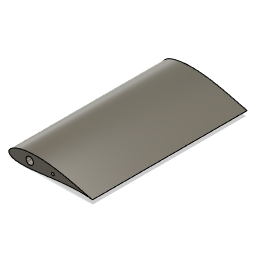
Joukowsky Refactor v1 (Autodesk Fusion 360 design; units mm, degrees)
Autodesk Fusion 360 part; units mm, degrees
sketch "Esquisse2" plane through (0, 0, 0) normal (0, 0, 1) x (1, 0, 0)
  spline S0 degree 5 poles (50, 0) (50, 0) (49.9928, 0.0013) (49.9605, 0.0071) (49.9137, 0.0157) (49.8549, 0.027) (49.7783, 0.0417) (49.6918, 0.0586) (49.6021, 0.0764) (49.5093, 0.0951) (49.4111, 0.1151) (49.3071, 0.1365) (49.1985, 0.159) (49.0867, 0.1824) (48.9721, 0.2067) (48.8543, 0.2319) (48.7333, 0.2579) (48.6092, 0.2848) (48.4821, 0.3126) (48.3526, 0.3411) (48.2206, 0.3703) (48.0864, 0.4002) (47.9499, 0.4309) (47.8111, 0.4622) (47.6702, 0.4942) (47.5272, 0.5268) (47.3822, 0.56) (47.2354, 0.5939) (47.0867, 0.6283) (46.9363, 0.6633) (46.7842, 0.6989) (46.6303, 0.735) (46.4749, 0.7717) (46.3178, 0.8089) (46.1592, 0.8466) (45.9991, 0.8848) (45.8376, 0.9234) (45.6746, 0.9626) (45.5102, 1.0022) (45.3445, 1.0423) (45.1775, 1.0828) (45.0092, 1.1238) (44.8396, 1.1652) (44.6688, 1.207) (44.4967, 1.2492) (44.3235, 1.2918) (44.1492, 1.3348) (43.9737, 1.3782) (43.797, 1.422) (43.6194, 1.4661) (43.4406, 1.5106) (43.2608, 1.5554) (43.08, 1.6006) (42.8981, 1.6461) (42.7153, 1.692) (42.5315, 1.7382) (42.3468, 1.7847) (42.1611, 1.8315) (41.9745, 1.8786) (41.787, 1.926) (41.5986, 1.9736) (41.4094, 2.0216) (41.2192, 2.0699) (41.0283, 2.1184) (40.8365, 2.1671) (40.6439, 2.2162) (40.4505, 2.2654) (40.2564, 2.315) (40.0614, 2.3647) (39.8657, 2.4147) (39.6692, 2.4649) (39.472, 2.5154) (39.2741, 2.566) (39.0754, 2.6169) (38.8761, 2.668) (38.676, 2.7192) (38.4753, 2.7707) (38.2738, 2.8223) (38.0718, 2.8742) (37.869, 2.9262) (37.6656, 2.9784) (37.4616, 3.0307) (37.257, 3.0832) (37.0517, 3.1359) (36.8458, 3.1887) (36.6394, 3.2417) (36.4323, 3.2948) (36.2247, 3.348) (36.0164, 3.4014) (35.8076, 3.4549) (35.5983, 3.5085) (35.3884, 3.5623) (35.1779, 3.6161) (34.9669, 3.6701) (34.7554, 3.7241) (34.5434, 3.7783) (34.3308, 3.8326) (34.1177, 3.8869) (33.9041, 3.9414) (33.6901, 3.9959) (33.4755, 4.0505) (33.2605, 4.1051) (33.0449, 4.1599) (32.8289, 4.2147) (32.6125, 4.2696) (32.3956, 4.3245) (32.1782, 4.3794) (31.9604, 4.4345) (31.7421, 4.4895) (31.5234, 4.5446) (31.3043, 4.5998) (31.0848, 4.6549) (30.8648, 4.7101) (30.6444, 4.7653) (30.4237, 4.8206) (30.2025, 4.8758) (29.9809, 4.9311) (29.7589, 4.9863) (29.5366, 5.0416) (29.3138, 5.0969) (29.0907, 5.1521) (28.8672, 5.2074) (28.6433, 5.2627) (28.4191, 5.3179) (28.1945, 5.3731) (27.9696, 5.4283) (27.7443, 5.4834) (27.5186, 5.5386) (27.2927, 5.5937) (27.0664, 5.6487) (26.8397, 5.7037) (26.6128, 5.7587) (26.3855, 5.8136) (26.1578, 5.8685) (25.9299, 5.9233) (25.7017, 5.9781) (25.4731, 6.0328) (25.2443, 6.0874) (25.0152, 6.142) (24.7857, 6.1965) (24.556, 6.2509) (24.326, 6.3052) (24.0957, 6.3595) (23.8651, 6.4136) (23.6342, 6.4677) (23.4031, 6.5217) (23.1717, 6.5756) (22.9401, 6.6293) (22.7081, 6.683) (22.476, 6.7366) (22.2435, 6.7901) (22.0109, 6.8434) (21.7779, 6.8967) (21.5448, 6.9498) (21.3114, 7.0028) (21.0777, 7.0556) (20.8438, 7.1084) (20.6097, 7.161) (20.3754, 7.2135) (20.1408, 7.2658) (19.9061, 7.318) (19.6711, 7.3701) (19.4359, 7.422) (19.2005, 7.4738) (18.9648, 7.5254) (18.729, 7.5768) (18.493, 7.6281) (18.2568, 7.6792) (18.0204, 7.7302) (17.7838, 7.781) (17.547, 7.8316) (17.31, 7.8821) (17.0728, 7.9324) (16.8355, 7.9825) (16.598, 8.0324) (16.3603, 8.0821) (16.1225, 8.1317) (15.8845, 8.181) (15.6463, 8.2302) (15.4079, 8.2791) (15.1694, 8.3279) (14.9308, 8.3765) (14.692, 8.4248) (14.453, 8.473) (14.2139, 8.5209) (13.9747, 8.5686) (13.7353, 8.6162) (13.4958, 8.6635) (13.2561, 8.7105) (13.0163, 8.7574) (12.7764, 8.804) (12.5364, 8.8504) (12.2962, 8.8966) (12.0559, 8.9425) (11.8155, 8.9882) (11.575, 9.0337) (11.3344, 9.0789) (11.0936, 9.1238) (10.8528, 9.1686) (10.6118, 9.213) (10.3708, 9.2572) (10.1296, 9.3012) (9.8884, 9.3449) (9.647, 9.3884) (9.4056, 9.4315) (9.1641, 9.4745) (8.9225, 9.5171) (8.6808, 9.5595) (8.439, 9.6016) (8.1972, 9.6434) (7.9553, 9.685) (7.7133, 9.7263) (7.4712, 9.7673) (7.2291, 9.808) (6.9869, 9.8484) (6.7447, 9.8886) (6.5023, 9.9284) (6.26, 9.968) (6.0176, 10.0072) (5.7751, 10.0462) (5.5326, 10.0848) (5.29, 10.1232) (5.0474, 10.1612) (4.8048, 10.199) (4.5621, 10.2364) (4.3194, 10.2735) (4.0766, 10.3103) (3.8338, 10.3468) (3.591, 10.383) (3.3482, 10.4188) (3.1053, 10.4543) (2.8624, 10.4895) (2.6196, 10.5244) (2.3766, 10.5589) (2.1337, 10.5931) (1.8908, 10.627) (1.6479, 10.6605) (1.4049, 10.6937) (1.162, 10.7265) (0.9191, 10.759) (0.6761, 10.7912) (0.4332, 10.823) (0.1903, 10.8545) (-0.0526, 10.8856) (-0.2955, 10.9163) (-0.5384, 10.9467) (-0.7812, 10.9768) (-1.024, 11.0065) (-1.2668, 11.0358) (-1.5096, 11.0647) (-1.7524, 11.0933) (-1.9951, 11.1215) (-2.2378, 11.1494) (-2.4804, 11.1768) (-2.723, 11.2039) (-2.9655, 11.2306) (-3.208, 11.257) (-3.4505, 11.2829) (-3.6929, 11.3085) (-3.9352, 11.3337) (-4.1775, 11.3585) (-4.4198, 11.3829) (-4.6619, 11.407) (-4.904, 11.4306) (-5.1461, 11.4538) (-5.388, 11.4767) (-5.6299, 11.4991) (-5.8717, 11.5211) (-6.1135, 11.5428) (-6.3551, 11.564) (-6.5967, 11.5848) (-6.8382, 11.6052) (-7.0796, 11.6252) (-7.3209, 11.6448) (-7.5621, 11.664) (-7.8032, 11.6828) (-8.0442, 11.7011) (-8.2851, 11.7191) (-8.5259, 11.7366) (-8.7665, 11.7536) (-9.0071, 11.7703) (-9.2476, 11.7865) (-9.4879, 11.8023) (-9.7281, 11.8177) (-9.9682, 11.8326) (-10.2081, 11.8471) (-10.448, 11.8612) (-10.6877, 11.8748) (-10.9272, 11.888) (-11.1666, 11.9008) (-11.4059, 11.9131) (-11.6451, 11.9249) (-11.884, 11.9364) (-12.1229, 11.9473) (-12.3616, 11.9578) (-12.6001, 11.9679) (-12.8384, 11.9775) (-13.0766, 11.9867) (-13.3147, 11.9954) (-13.5525, 12.0036) (-13.7902, 12.0114) (-14.0278, 12.0187) (-14.2651, 12.0256) (-14.5022, 12.032) (-14.7392, 12.0379) (-14.976, 12.0433) (-15.2126, 12.0483) (-15.449, 12.0528) (-15.6852, 12.0569) (-15.9212, 12.0604) (-16.157, 12.0635) (-16.3926, 12.0661) (-16.6279, 12.0682) (-16.8631, 12.0699) (-17.0981, 12.071) (-17.3328, 12.0717) (-17.5673, 12.0719) (-17.8016, 12.0716) (-18.0356, 12.0708) (-18.2694, 12.0695) (-18.503, 12.0678) (-18.7363, 12.0655) (-18.9694, 12.0627) (-19.2022, 12.0595) (-19.4348, 12.0557) (-19.6672, 12.0515) (-19.8992, 12.0467) (-20.131, 12.0414) (-20.3626, 12.0357) (-20.5939, 12.0294) (-20.8249, 12.0226) (-21.0556, 12.0153) (-21.286, 12.0075) (-21.5162, 11.9992) (-21.7461, 11.9904) (-21.9757, 11.981) (-22.205, 11.9711) (-22.4339, 11.9608) (-22.6626, 11.9499) (-22.891, 11.9384) (-23.1191, 11.9265) (-23.3468, 11.914) (-23.5743, 11.901) (-23.8014, 11.8875) (-24.0282, 11.8734) (-24.2546, 11.8588) (-24.4808, 11.8437) (-24.7065, 11.8281) (-24.932, 11.8119) (-25.1571, 11.7952) (-25.3818, 11.7779) (-25.6062, 11.7601) (-25.8302, 11.7418) (-26.0539, 11.7229) (-26.2772, 11.7035) (-26.5001, 11.6835) (-26.7227, 11.663) (-26.9448, 11.6419) (-27.1666, 11.6203) (-27.388, 11.5981) (-27.609, 11.5754) (-27.8296, 11.5522) (-28.0498, 11.5284) (-28.2696, 11.504) (-28.489, 11.479) (-28.7079, 11.4536) (-28.9265, 11.4275) (-29.1446, 11.4009) (-29.3622, 11.3737) (-29.5795, 11.346) (-29.7963, 11.3177) (-30.0126, 11.2888) (-30.2285, 11.2594) (-30.444, 11.2294) (-30.6589, 11.1988) (-30.8734, 11.1676) (-31.0875, 11.1359) (-31.301, 11.1036) (-31.5141, 11.0707) (-31.7267, 11.0373) (-31.9388, 11.0033) (-32.1504, 10.9686) (-32.3615, 10.9334) (-32.5721, 10.8977) (-32.7821, 10.8613) (-32.9917, 10.8244) (-33.2007, 10.7868) (-33.4092, 10.7487) (-33.6171, 10.71) (-33.8245, 10.6707) (-34.0313, 10.6308) (-34.2376, 10.5903) (-34.4433, 10.5492) (-34.6485, 10.5075) (-34.8531, 10.4653) (-35.0571, 10.4224) (-35.2605, 10.3789) (-35.4633, 10.3348) (-35.6655, 10.2901) (-35.8671, 10.2448) (-36.0681, 10.1989) (-36.2684, 10.1524) (-36.4681, 10.1053) (-36.6672, 10.0576) (-36.8657, 10.0093) (-37.0635, 9.9603) (-37.2606, 9.9107) (-37.4571, 9.8606) (-37.6529, 9.8097) (-37.848, 9.7583) (-38.0424, 9.7063) (-38.2361, 9.6536) (-38.4292, 9.6003) (-38.6215, 9.5464) (-38.8131, 9.4919) (-39.0039, 9.4367) (-39.1941, 9.3809) (-39.3834, 9.3245) (-39.572, 9.2674) (-39.7599, 9.2097) (-39.947, 9.1514) (-40.1333, 9.0924) (-40.3188, 9.0328) (-40.5035, 8.9726) (-40.6874, 8.9117) (-40.8705, 8.8501) (-41.0527, 8.7879) (-41.2341, 8.7251) (-41.4146, 8.6616) (-41.5943, 8.5975) (-41.7731, 8.5327) (-41.9511, 8.4673) (-42.1281, 8.4012) (-42.3042, 8.3344) (-42.4795, 8.267) (-42.6537, 8.1989) (-42.8271, 8.1302) (-42.9995, 8.0608) (-43.1709, 7.9907) (-43.3413, 7.9199) (-43.5108, 7.8485) (-43.6793, 7.7764) (-43.8467, 7.7037) (-44.0131, 7.6302) (-44.1784, 7.5561) (-44.3427, 7.4813) (-44.5059, 7.4058) (-44.6681, 7.3296) (-44.8291, 7.2528) (-44.989, 7.1752) (-45.1478, 7.097) (-45.3054, 7.018) (-45.4618, 6.9384) (-45.6171, 6.8581) (-45.7711, 6.777) (-45.9239, 6.6953) (-46.0755, 6.6128) (-46.2258, 6.5297) (-46.3748, 6.4458) (-46.5226, 6.3612) (-46.669, 6.2759) (-46.814, 6.1899) (-46.9577, 6.1031) (-47.1, 6.0157) (-47.2409, 5.9275) (-47.3804, 5.8385) (-47.5184, 5.7489) (-47.6549, 5.6585) (-47.7899, 5.5674) (-47.9233, 5.4755) (-48.0552, 5.3829) (-48.1855, 5.2895) (-48.3141, 5.1954) (-48.4411, 5.1005) (-48.5664, 5.0049) (-48.69, 4.9086) (-48.8118, 4.8114) (-48.9319, 4.7135) (-49.0501, 4.6149) (-49.1664, 4.5155) (-49.2808, 4.4153) (-49.3933, 4.3144) (-49.5038, 4.2127) (-49.6123, 4.1102) (-49.7187, 4.0069) (-49.823, 3.9029) (-49.9251, 3.7981) (-50.0249, 3.6926) (-50.1225, 3.5862) (-50.2178, 3.4791) (-50.3107, 3.3713) (-50.4011, 3.2627) (-50.4891, 3.1533) (-50.5744, 3.0432) (-50.6572, 2.9323) (-50.7372, 2.8207) (-50.8145, 2.7084) (-50.8889, 2.5954) (-50.9604, 2.4817) (-51.0289, 2.3673) (-51.0943, 2.2522) (-51.1566, 2.1365) (-51.2157, 2.0202) (-51.2714, 1.9033) (-51.3238, 1.7858) (-51.3726, 1.6679) (-51.4179, 1.5494) (-51.4594, 1.4305) (-51.4973, 1.3111) (-51.5313, 1.1915) (-51.5613, 1.0715) (-51.5873, 0.9514) (-51.6093, 0.831) (-51.6271, 0.7106) (-51.6406, 0.5902) (-51.6498, 0.4699) (-51.6547, 0.3498) (-51.6551, 0.2299) (-51.6511, 0.1103) (-51.6427, -0.0088) (-51.6297, -0.1273) (-51.6122, -0.2452) (-51.5902, -0.3623) (-51.5638, -0.4786) (-51.5328, -0.594) (-51.4975, -0.7084) (-51.4577, -0.8216) (-51.4137, -0.9336) (-51.3654, -1.0444) (-51.3129, -1.1538) (-51.2563, -1.2619) (-51.1956, -1.3684) (-51.1311, -1.4735) (-51.0627, -1.5771) (-50.9906, -1.679) (-50.9148, -1.7794) (-50.8355, -1.8781) (-50.7527, -1.9752) (-50.6666, -2.0706) (-50.5772, -2.1643) (-50.4847, -2.2564) (-50.389, -2.3468) (-50.2904, -2.4355) (-50.1889, -2.5226) (-50.0846, -2.608) (-49.9776, -2.6918) (-49.8679, -2.774) (-49.7557, -2.8545) (-49.6409, -2.9334) (-49.5237, -3.0108) (-49.4041, -3.0866) (-49.2823, -3.1609) (-49.1582, -3.2336) (-49.0319, -3.3048) (-48.9035, -3.3745) (-48.773, -3.4428) (-48.6405, -3.5096) (-48.5061, -3.575) (-48.3697, -3.639) (-48.2314, -3.7017) (-48.0914, -3.7629) (-47.9495, -3.8228) (-47.8059, -3.8814) (-47.6606, -3.9386) (-47.5136, -3.9946) (-47.365, -4.0493) (-47.2148, -4.1028) (-47.063, -4.155) (-46.9097, -4.206) (-46.7549, -4.2558) (-46.5987, -4.3044) (-46.4409, -4.3518) (-46.2818, -4.3981) (-46.1213, -4.4433) (-45.9594, -4.4874) (-45.7962, -4.5303) (-45.6317, -4.5722) (-45.4659, -4.6129) (-45.2988, -4.6527) (-45.1305, -4.6913) (-44.9609, -4.729) (-44.7902, -4.7656) (-44.6182, -4.8012) (-44.4451, -4.8359) (-44.2709, -4.8695) (-44.0955, -4.9022) (-43.919, -4.934) (-43.7414, -4.9648) (-43.5628, -4.9946) (-43.383, -5.0236) (-43.2023, -5.0516) (-43.0205, -5.0787) (-42.8377, -5.105) (-42.6538, -5.1304) (-42.469, -5.1549) (-42.2833, -5.1786) (-42.0965, -5.2014) (-41.9088, -5.2234) (-41.7202, -5.2445) (-41.5307, -5.2649) (-41.3402, -5.2844) (-41.1489, -5.3032) (-40.9566, -5.3212) (-40.7635, -5.3384) (-40.5696, -5.3548) (-40.3747, -5.3705) (-40.179, -5.3854) (-39.9825, -5.3995) (-39.7852, -5.413) (-39.587, -5.4257) (-39.3881, -5.4377) (-39.1883, -5.449) (-38.9878, -5.4596) (-38.7865, -5.4695) (-38.5844, -5.4787) (-38.3816, -5.4872) (-38.178, -5.4951) (-37.9736, -5.5023) (-37.7686, -5.5088) (-37.5628, -5.5147) (-37.3562, -5.52) (-37.149, -5.5246) (-36.9411, -5.5286) (-36.7325, -5.532) (-36.5231, -5.5348) (-36.3131, -5.5369) (-36.1025, -5.5385) (-35.8911, -5.5395) (-35.6791, -5.5398) (-35.4665, -5.5396) (-35.2532, -5.5389) (-35.0392, -5.5375) (-34.8246, -5.5356) (-34.6094, -5.5332) (-34.3936, -5.5302) (-34.1772, -5.5266) (-33.9601, -5.5225) (-33.7425, -5.5179) (-33.5242, -5.5128) (-33.3053, -5.5071) (-33.0859, -5.501) (-32.8659, -5.4943) (-32.6453, -5.4871) (-32.4241, -5.4794) (-32.2024, -5.4713) (-31.9801, -5.4626) (-31.7573, -5.4535) (-31.5339, -5.4439) (-31.31, -5.4338) (-31.0855, -5.4233) (-30.8605, -5.4123) (-30.6349, -5.4009) (-30.4089, -5.389) (-30.1823, -5.3767) (-29.9552, -5.3639) (-29.7276, -5.3507) (-29.4995, -5.3371) (-29.2709, -5.3231) (-29.0418, -5.3086) (-28.8122, -5.2938) (-28.5821, -5.2785) (-28.3515, -5.2628) (-28.1204, -5.2468) (-27.8889, -5.2303) (-27.6569, -5.2135) (-27.4245, -5.1962) (-27.1915, -5.1786) (-26.9582, -5.1607) (-26.7243, -5.1423) (-26.4901, -5.1237) (-26.2553, -5.1046) (-26.0202, -5.0852) (-25.7846, -5.0655) (-25.5485, -5.0454) (-25.312, -5.0249) (-25.0752, -5.0042) (-24.8378, -4.9831) (-24.6001, -4.9617) (-24.362, -4.9399) (-24.1234, -4.9179) (-23.8844, -4.8955) (-23.6451, -4.8728) (-23.4053, -4.8499) (-23.1651, -4.8266) (-22.9246, -4.803) (-22.6836, -4.7792) (-22.4423, -4.7551) (-22.2006, -4.7307) (-21.9585, -4.706) (-21.7161, -4.681) (-21.4732, -4.6558) (-21.23, -4.6303) (-20.9865, -4.6046) (-20.7426, -4.5786) (-20.4983, -4.5523) (-20.2536, -4.5258) (-20.0087, -4.4991) (-19.7633, -4.4722) (-19.5177, -4.445) (-19.2716, -4.4175) (-19.0253, -4.3899) (-18.7786, -4.362) (-18.5316, -4.3339) (-18.2843, -4.3056) (-18.0366, -4.2771) (-17.7886, -4.2484) (-17.5403, -4.2195) (-17.2917, -4.1904) (-17.0428, -4.1611) (-16.7935, -4.1316) (-16.544, -4.1019) (-16.2942, -4.0721) (-16.044, -4.0421) (-15.7936, -4.0119) (-15.5429, -3.9815) (-15.2919, -3.951) (-15.0406, -3.9203) (-14.789, -3.8895) (-14.5372, -3.8585) (-14.285, -3.8274) (-14.0326, -3.7961) (-13.78, -3.7646) (-13.527, -3.7331) (-13.2738, -3.7014) (-13.0204, -3.6696) (-12.7667, -3.6376) (-12.5127, -3.6056) (-12.2585, -3.5734) (-12.004, -3.5411) (-11.7493, -3.5087) (-11.4944, -3.4762) (-11.2392, -3.4436) (-10.9838, -3.4109) (-10.7281, -3.3781) (-10.4722, -3.3452) (-10.2161, -3.3122) (-9.9598, -3.2792) (-9.7033, -3.246) (-9.4465, -3.2128) (-9.1895, -3.1795) (-8.9324, -3.1462) (-8.675, -3.1128) (-8.4174, -3.0793) (-8.1596, -3.0457) (-7.9016, -3.0122) (-7.6434, -2.9785) (-7.385, -2.9448) (-7.1265, -2.9111) (-6.8677, -2.8773) (-6.6088, -2.8435) (-6.3497, -2.8097) (-6.0905, -2.7758) (-5.831, -2.742) (-5.5714, -2.708) (-5.3116, -2.6741) (-5.0517, -2.6402) (-4.7916, -2.6062) (-4.5313, -2.5723) (-4.2709, -2.5383) (-4.0104, -2.5044) (-3.7497, -2.4704) (-3.4888, -2.4364) (-3.2279, -2.4025) (-2.9667, -2.3686) (-2.7055, -2.3347) (-2.4441, -2.3008) (-2.1826, -2.2669) (-1.921, -2.2331) (-1.6593, -2.1993) (-1.3974, -2.1655) (-1.1354, -2.1318) (-0.8734, -2.0981) (-0.6112, -2.0644) (-0.3489, -2.0308) (-0.0865, -1.9973) (0.1759, -1.9638) (0.4385, -1.9303) (0.7012, -1.897) (0.9639, -1.8636) (1.2267, -1.8304) (1.4896, -1.7972) (1.7526, -1.7641) (2.0156, -1.7311) (2.2787, -1.6982) (2.5419, -1.6653) (2.8051, -1.6325) (3.0684, -1.5999) (3.3317, -1.5673) (3.5951, -1.5348) (3.8585, -1.5024) (4.122, -1.4701) (4.3855, -1.4379) (4.649, -1.4058) (4.9126, -1.3739) (5.1762, -1.342) (5.4398, -1.3103) (5.7034, -1.2787) (5.9671, -1.2472) (6.2307, -1.2159) (6.4944, -1.1846) (6.758, -1.1536) (7.0217, -1.1226) (7.2854, -1.0918) (7.549, -1.0611) (7.8126, -1.0306) (8.0763, -1.0002) (8.3398, -0.97) (8.6034, -0.9399) (8.867, -0.91) (9.1305, -0.8803) (9.3939, -0.8507) (9.6574, -0.8213) (9.9207, -0.792) (10.1841, -0.7629) (10.4473, -0.734) (10.7105, -0.7053) (10.9737, -0.6768) (11.2368, -0.6484) (11.4998, -0.6202) (11.7627, -0.5922) (12.0256, -0.5644) (12.2883, -0.5368) (12.551, -0.5094) (12.8136, -0.4822) (13.0761, -0.4552) (13.3385, -0.4284) (13.6007, -0.4018) (13.8629, -0.3754) (14.1249, -0.3493) (14.3868, -0.3233) (14.6486, -0.2976) (14.9103, -0.2721) (15.1718, -0.2468) (15.4332, -0.2217) (15.6944, -0.1969) (15.9555, -0.1723) (16.2164, -0.1479) (16.4772, -0.1238) (16.7378, -0.0999) (16.9982, -0.0762) (17.2584, -0.0528) (17.5185, -0.0296) (17.7784, -0.0067) (18.0381, 0.016) (18.2976, 0.0384) (18.5568, 0.0606) (18.8159, 0.0825) (19.0748, 0.1041) (19.3334, 0.1255) (19.5918, 0.1466) (19.85, 0.1675) (20.108, 0.1881) (20.3657, 0.2084) (20.6232, 0.2285) (20.8804, 0.2482) (21.1373, 0.2677) (21.394, 0.2869) (21.6504, 0.3059) (21.9066, 0.3245) (22.1624, 0.3429) (22.418, 0.361) (22.6733, 0.3788) (22.9282, 0.3963) (23.1829, 0.4135) (23.4373, 0.4304) (23.6913, 0.4471) (23.945, 0.4634) (24.1984, 0.4794) (24.4514, 0.4952) (24.7041, 0.5106) (24.9564, 0.5257) (25.2084, 0.5405) (25.46, 0.555) (25.7113, 0.5692) (25.9621, 0.5831) (26.2126, 0.5967) (26.4627, 0.61) (26.7124, 0.6229) (26.9617, 0.6355) (27.2105, 0.6479) (27.459, 0.6599) (27.707, 0.6715) (27.9546, 0.6829) (28.2017, 0.6939) (28.4484, 0.7046) (28.6946, 0.715) (28.9404, 0.725) (29.1856, 0.7348) (29.4304, 0.7441) (29.6747, 0.7532) (29.9186, 0.7619) (30.1619, 0.7703) (30.4046, 0.7784) (30.6469, 0.7861) (30.8886, 0.7935) (31.1298, 0.8006) (31.3705, 0.8073) (31.6105, 0.8137) (31.8501, 0.8198) (32.089, 0.8255) (32.3273, 0.8308) (32.5651, 0.8359) (32.8023, 0.8406) (33.0388, 0.8449) (33.2747, 0.8489) (33.51, 0.8526) (33.7446, 0.8559) (33.9786, 0.8589) (34.212, 0.8616) (34.4446, 0.8639) (34.6766, 0.8658) (34.9079, 0.8674) (35.1384, 0.8687) (35.3683, 0.8696) (35.5974, 0.8702) (35.8258, 0.8705) (36.0535, 0.8704) (36.2803, 0.87) (36.5065, 0.8692) (36.7318, 0.8681) (36.9563, 0.8666) (37.18, 0.8648) (37.4029, 0.8627) (37.625, 0.8602) (37.8462, 0.8574) (38.0666, 0.8543) (38.2861, 0.8508) (38.5047, 0.847) (38.7224, 0.8428) (38.9392, 0.8383) (39.155, 0.8335) (39.3699, 0.8284) (39.5839, 0.8229) (39.7969, 0.8171) (40.0088, 0.811) (40.2198, 0.8045) (40.4298, 0.7978) (40.6387, 0.7907) (40.8466, 0.7833) (41.0534, 0.7756) (41.2591, 0.7675) (41.4637, 0.7592) (41.6671, 0.7505) (41.8694, 0.7416) (42.0706, 0.7323) (42.2706, 0.7228) (42.4693, 0.7129) (42.6668, 0.7028) (42.8631, 0.6923) (43.0581, 0.6816) (43.2518, 0.6706) (43.4442, 0.6593) (43.6353, 0.6477) (43.825, 0.6359) (44.0132, 0.6238) (44.2001, 0.6114) (44.3855, 0.5988) (44.5695, 0.5859) (44.7519, 0.5728) (44.9328, 0.5595) (45.1121, 0.5459) (45.2898, 0.532) (45.4658, 0.518) (45.6402, 0.5037) (45.8129, 0.4893) (45.9838, 0.4746) (46.153, 0.4597) (46.3203, 0.4447) (46.4857, 0.4294) (46.6491, 0.414) (46.8106, 0.3985) (46.97, 0.3828) (47.1273, 0.367) (47.2826, 0.351) (47.4356, 0.3349) (47.5863, 0.3187) (47.7346, 0.3025) (47.8804, 0.2862) (48.0237, 0.2698) (48.1644, 0.2534) (48.3024, 0.237) (48.4378, 0.2206) (48.5702, 0.2042) (48.6994, 0.1879) (48.825, 0.1717) (48.9471, 0.1557) (49.0659, 0.1397) (49.1815, 0.1239) (49.2934, 0.1083) (49.4003, 0.093) (49.5009, 0.0784) (49.596, 0.0644) (49.6878, 0.0504) (49.776, 0.0366) (49.8535, 0.0243) (49.913, 0.0148) (49.9605, 0.0068) (49.9928, 0.0012) (50, 0) (50, 0) knots 0 0 0 0 0 0 0.00100503 0.00201005 0.00301508 0.0040201 0.00502513 0.00603015 0.00703518 0.0080402 0.00904523 0.01005025 0.01105528 0.0120603 0.01306533 0.01407035 0.01507538 0.0160804 0.01708543 0.01809045 0.01909548 0.0201005 0.02110553 0.02211055 0.02311558 0.0241206 0.02512563 0.02613065 0.02713568 0.0281407 0.02914573 0.03015075 0.03115578 0.0321608 0.03316583 0.03417085 0.03517588 0.0361809 0.03718593 0.03819095 0.03919598 0.04020101 0.04120603 0.04221106 0.04321608 0.04422111 0.04522613 0.04623116 0.04723618 0.04824121 0.04924623 0.05025126 0.05125628 0.05226131 0.05326633 0.05427136 0.05527638 0.05628141 0.05728643 0.05829146 0.05929648 0.06030151 0.06130653 0.06231156 0.06331658 0.06432161 0.06532663 0.06633166 0.06733668 0.06834171 0.06934673 0.07035176 0.07135678 0.07236181 0.07336683 0.07437186 0.07537688 0.07638191 0.07738693 0.07839196 0.07939698 0.08040201 0.08140704 0.08241206 0.08341709 0.08442211 0.08542714 0.08643216 0.08743719 0.08844221 0.08944724 0.09045226 0.09145729 0.09246231 0.09346734 0.09447236 0.09547739 0.09648241 0.09748744 0.09849246 0.09949749 0.10050251 0.10150754 0.10251256 0.10351759 0.10452261 0.10552764 0.10653266 0.10753769 0.10854271 0.10954774 0.11055276 0.11155779 0.11256281 0.11356784 0.11457286 0.11557789 0.11658291 0.11758794 0.11859296 0.11959799 0.12060302 0.12160804 0.12261307 0.12361809 0.12462312 0.12562814 0.12663317 0.12763819 0.12864322 0.12964824 0.13065327 0.13165829 0.13266332 0.13366834 0.13467337 0.13567839 0.13668342 0.13768844 0.13869347 0.13969849 0.14070352 0.14170854 0.14271357 0.14371859 0.14472362 0.14572864 0.14673367 0.14773869 0.14874372 0.14974874 0.15075377 0.15175879 0.15276382 0.15376884 0.15477387 0.15577889 0.15678392 0.15778894 0.15879397 0.15979899 0.16080402 0.16180905 0.16281407 0.1638191 0.16482412 0.16582915 0.16683417 0.1678392 0.16884422 0.16984925 0.17085427 0.1718593 0.17286432 0.17386935 0.17487437 0.1758794 0.17688442 0.17788945 0.17889447 0.1798995 0.18090452 0.18190955 0.18291457 0.1839196 0.18492462 0.18592965 0.18693467 0.1879397 0.18894472 0.18994975 0.19095477 0.1919598 0.19296482 0.19396985 0.19497487 0.1959799 0.19698492 0.19798995 0.19899497 0.2 0.20100503 0.20201005 0.20301508 0.2040201 0.20502513 0.20603015 0.20703518 0.2080402 0.20904523 0.21005025 0.21105528 0.2120603 0.21306533 0.21407035 0.21507538 0.2160804 0.21708543 0.21809045 0.21909548 0.2201005 0.22110553 0.22211055 0.22311558 0.2241206 0.22512563 0.22613065 0.22713568 0.2281407 0.22914573 0.23015075 0.23115578 0.2321608 0.23316583 0.23417085 0.23517588 0.2361809 0.23718593 0.23819095 0.23919598 0.24020101 0.24120603 0.24221106 0.24321608 0.24422111 0.24522613 0.24623116 0.24723618 0.24824121 0.24924623 0.25025126 0.25125628 0.25226131 0.25326633 0.25427136 0.25527638 0.25628141 0.25728643 0.25829146 0.25929648 0.26030151 0.26130653 0.26231156 0.26331658 0.26432161 0.26532663 0.26633166 0.26733668 0.26834171 0.26934673 0.27035176 0.27135678 0.27236181 0.27336683 0.27437186 0.27537688 0.27638191 0.27738693 0.27839196 0.27939698 0.28040201 0.28140704 0.28241206 0.28341709 0.28442211 0.28542714 0.28643216 0.28743719 0.28844221 0.28944724 0.29045226 0.29145729 0.29246231 0.29346734 0.29447236 0.29547739 0.29648241 0.29748744 0.29849246 0.29949749 0.30050251 0.30150754 0.30251256 0.30351759 0.30452261 0.30552764 0.30653266 0.30753769 0.30854271 0.30954774 0.31055276 0.31155779 0.31256281 0.31356784 0.31457286 0.31557789 0.31658291 0.31758794 0.31859296 0.31959799 0.32060302 0.32160804 0.32261307 0.32361809 0.32462312 0.32562814 0.32663317 0.32763819 0.32864322 0.32964824 0.33065327 0.33165829 0.33266332 0.33366834 0.33467337 0.33567839 0.33668342 0.33768844 0.33869347 0.33969849 0.34070352 0.34170854 0.34271357 0.34371859 0.34472362 0.34572864 0.34673367 0.34773869 0.34874372 0.34974874 0.35075377 0.35175879 0.35276382 0.35376884 0.35477387 0.35577889 0.35678392 0.35778894 0.35879397 0.35979899 0.36080402 0.36180905 0.36281407 0.3638191 0.36482412 0.36582915 0.36683417 0.3678392 0.36884422 0.36984925 0.37085427 0.3718593 0.37286432 0.37386935 0.37487437 0.3758794 0.37688442 0.37788945 0.37889447 0.3798995 0.38090452 0.38190955 0.38291457 0.3839196 0.38492462 0.38592965 0.38693467 0.3879397 0.38894472 0.38994975 0.39095477 0.3919598 0.39296482 0.39396985 0.39497487 0.3959799 0.39698492 0.39798995 0.39899497 0.4 0.40100503 0.40201005 0.40301508 0.4040201 0.40502513 0.40603015 0.40703518 0.4080402 0.40904523 0.41005025 0.41105528 0.4120603 0.41306533 0.41407035 0.41507538 0.4160804 0.41708543 0.41809045 0.41909548 0.4201005 0.42110553 0.42211055 0.42311558 0.4241206 0.42512563 0.42613065 0.42713568 0.4281407 0.42914573 0.43015075 0.43115578 0.4321608 0.43316583 0.43417085 0.43517588 0.4361809 0.43718593 0.43819095 0.43919598 0.44020101 0.44120603 0.44221106 0.44321608 0.44422111 0.44522613 0.44623116 0.44723618 0.44824121 0.44924623 0.45025126 0.45125628 0.45226131 0.45326633 0.45427136 0.45527638 0.45628141 0.45728643 0.45829146 0.45929648 0.46030151 0.46130653 0.46231156 0.46331658 0.46432161 0.46532663 0.46633166 0.46733668 0.46834171 0.46934673 0.47035176 0.47135678 0.47236181 0.47336683 0.47437186 0.47537688 0.47638191 0.47738693 0.47839196 0.47939698 0.48040201 0.48140704 0.48241206 0.48341709 0.48442211 0.48542714 0.48643216 0.48743719 0.48844221 0.48944724 0.49045226 0.49145729 0.49246231 0.49346734 0.49447236 0.49547739 0.49648241 0.49748744 0.49849246 0.49949749 0.50050251 0.50150754 0.50251256 0.50351759 0.50452261 0.50552764 0.50653266 0.50753769 0.50854271 0.50954774 0.51055276 0.51155779 0.51256281 0.51356784 0.51457286 0.51557789 0.51658291 0.51758794 0.51859296 0.51959799 0.52060302 0.52160804 0.52261307 0.52361809 0.52462312 0.52562814 0.52663317 0.52763819 0.52864322 0.52964824 0.53065327 0.53165829 0.53266332 0.53366834 0.53467337 0.53567839 0.53668342 0.53768844 0.53869347 0.53969849 0.54070352 0.54170854 0.54271357 0.54371859 0.54472362 0.54572864 0.54673367 0.54773869 0.54874372 0.54974874 0.55075377 0.55175879 0.55276382 0.55376884 0.55477387 0.55577889 0.55678392 0.55778894 0.55879397 0.55979899 0.56080402 0.56180905 0.56281407 0.5638191 0.56482412 0.56582915 0.56683417 0.5678392 0.56884422 0.56984925 0.57085427 0.5718593 0.57286432 0.57386935 0.57487437 0.5758794 0.57688442 0.57788945 0.57889447 0.5798995 0.58090452 0.58190955 0.58291457 0.5839196 0.58492462 0.58592965 0.58693467 0.5879397 0.58894472 0.58994975 0.59095477 0.5919598 0.59296482 0.59396985 0.59497487 0.5959799 0.59698492 0.59798995 0.59899497 0.6 0.60100503 0.60201005 0.60301508 0.6040201 0.60502513 0.60603015 0.60703518 0.6080402 0.60904523 0.61005025 0.61105528 0.6120603 0.61306533 0.61407035 0.61507538 0.6160804 0.61708543 0.61809045 0.61909548 0.6201005 0.62110553 0.62211055 0.62311558 0.6241206 0.62512563 0.62613065 0.62713568 0.6281407 0.62914573 0.63015075 0.63115578 0.6321608 0.63316583 0.63417085 0.63517588 0.6361809 0.63718593 0.63819095 0.63919598 0.64020101 0.64120603 0.64221106 0.64321608 0.64422111 0.64522613 0.64623116 0.64723618 0.64824121 0.64924623 0.65025126 0.65125628 0.65226131 0.65326633 0.65427136 0.65527638 0.65628141 0.65728643 0.65829146 0.65929648 0.66030151 0.66130653 0.66231156 0.66331658 0.66432161 0.66532663 0.66633166 0.66733668 0.66834171 0.66934673 0.67035176 0.67135678 0.67236181 0.67336683 0.67437186 0.67537688 0.67638191 0.67738693 0.67839196 0.67939698 0.68040201 0.68140704 0.68241206 0.68341709 0.68442211 0.68542714 0.68643216 0.68743719 0.68844221 0.68944724 0.69045226 0.69145729 0.69246231 0.69346734 0.69447236 0.69547739 0.69648241 0.69748744 0.69849246 0.69949749 0.70050251 0.70150754 0.70251256 0.70351759 0.70452261 0.70552764 0.70653266 0.70753769 0.70854271 0.70954774 0.71055276 0.71155779 0.71256281 0.71356784 0.71457286 0.71557789 0.71658291 0.71758794 0.71859296 0.71959799 0.72060302 0.72160804 0.72261307 0.72361809 0.72462312 0.72562814 0.72663317 0.72763819 0.72864322 0.72964824 0.73065327 0.73165829 0.73266332 0.73366834 0.73467337 0.73567839 0.73668342 0.73768844 0.73869347 0.73969849 0.74070352 0.74170854 0.74271357 0.74371859 0.74472362 0.74572864 0.74673367 0.74773869 0.74874372 0.74974874 0.75075377 0.75175879 0.75276382 0.75376884 0.75477387 0.75577889 0.75678392 0.75778894 0.75879397 0.75979899 0.76080402 0.76180905 0.76281407 0.7638191 0.76482412 0.76582915 0.76683417 0.7678392 0.76884422 0.76984925 0.77085427 0.7718593 0.77286432 0.77386935 0.77487437 0.7758794 0.77688442 0.77788945 0.77889447 0.7798995 0.78090452 0.78190955 0.78291457 0.7839196 0.78492462 0.78592965 0.78693467 0.7879397 0.78894472 0.78994975 0.79095477 0.7919598 0.79296482 0.79396985 0.79497487 0.7959799 0.79698492 0.79798995 0.79899497 0.8 0.80100503 0.80201005 0.80301508 0.8040201 0.80502513 0.80603015 0.80703518 0.8080402 0.80904523 0.81005025 0.81105528 0.8120603 0.81306533 0.81407035 0.81507538 0.8160804 0.81708543 0.81809045 0.81909548 0.8201005 0.82110553 0.82211055 0.82311558 0.8241206 0.82512563 0.82613065 0.82713568 0.8281407 0.82914573 0.83015075 0.83115578 0.8321608 0.83316583 0.83417085 0.83517588 0.8361809 0.83718593 0.83819095 0.83919598 0.84020101 0.84120603 0.84221106 0.84321608 0.84422111 0.84522613 0.84623116 0.84723618 0.84824121 0.84924623 0.85025126 0.85125628 0.85226131 0.85326633 0.85427136 0.85527638 0.85628141 0.85728643 0.85829146 0.85929648 0.86030151 0.86130653 0.86231156 0.86331658 0.86432161 0.86532663 0.86633166 0.86733668 0.86834171 0.86934673 0.87035176 0.87135678 0.87236181 0.87336683 0.87437186 0.87537688 0.87638191 0.87738693 0.87839196 0.87939698 0.88040201 0.88140704 0.88241206 0.88341709 0.88442211 0.88542714 0.88643216 0.88743719 0.88844221 0.88944724 0.89045226 0.89145729 0.89246231 0.89346734 0.89447236 0.89547739 0.89648241 0.89748744 0.89849246 0.89949749 0.90050251 0.90150754 0.90251256 0.90351759 0.90452261 0.90552764 0.90653266 0.90753769 0.90854271 0.90954774 0.91055276 0.91155779 0.91256281 0.91356784 0.91457286 0.91557789 0.91658291 0.91758794 0.91859296 0.91959799 0.92060302 0.92160804 0.92261307 0.92361809 0.92462312 0.92562814 0.92663317 0.92763819 0.92864322 0.92964824 0.93065327 0.93165829 0.93266332 0.93366834 0.93467337 0.93567839 0.93668342 0.93768844 0.93869347 0.93969849 0.94070352 0.94170854 0.94271357 0.94371859 0.94472362 0.94572864 0.94673367 0.94773869 0.94874372 0.94974874 0.95075377 0.95175879 0.95276382 0.95376884 0.95477387 0.95577889 0.95678392 0.95778894 0.95879397 0.95979899 0.96080402 0.96180905 0.96281407 0.9638191 0.96482412 0.96582915 0.96683417 0.9678392 0.96884422 0.96984925 0.97085427 0.9718593 0.97286432 0.97386935 0.97487437 0.9758794 0.97688442 0.97788945 0.97889447 0.9798995 0.98090452 0.98190955 0.98291457 0.9839196 0.98492462 0.98592965 0.98693467 0.9879397 0.98894472 0.98994975 0.99095477 0.9919598 0.99296482 0.99396985 0.99497487 0.9959799 0.99698492 0.99798995 0.99899497 1 1 1 1 1 1
  circle A0 centre (-26.2397, 3) radius 4.5
  line L0 (-58, 0) -> (59, 0) construction
  line L1 (-26.2397, 3) -> (1.7603, 3) construction
  circle A1 centre (1.7603, 3) radius 1.65
  point P0 (49.9677, 0.0059)
  point P1 (49.8713, 0.0239)
  point P2 (49.7117, 0.0548)
  point P3 (49.4901, 0.099)
  point P4 (49.2075, 0.1572)
  point P5 (48.8652, 0.2296)
  point P6 (48.4645, 0.3165)
  point P7 (48.0066, 0.4182)
  point P8 (47.4932, 0.5346)
  point P9 (46.9256, 0.6659)
  point P10 (46.3053, 0.8119)
  point P11 (45.6339, 0.9724)
  point P12 (44.913, 1.1472)
  point P13 (44.1443, 1.336)
  point P14 (43.3292, 1.5384)
  point P15 (42.4695, 1.7538)
  point P16 (41.5668, 1.9817)
  point P17 (40.6228, 2.2215)
  point P18 (39.6391, 2.4726)
  point P19 (38.6174, 2.7343)
  point P20 (37.5592, 3.0057)
  point P21 (36.4662, 3.2861)
  point P22 (35.34, 3.5746)
  point P23 (34.1823, 3.8705)
  point P24 (32.9945, 4.1727)
  point P25 (31.7783, 4.4804)
  point P26 (30.5352, 4.7927)
  point P27 (29.2667, 5.1085)
  point P28 (27.9743, 5.4271)
  point P29 (26.6595, 5.7474)
  point P30 (25.3237, 6.0684)
  point P31 (23.9685, 6.3893)
  point P32 (22.5952, 6.7091)
  point P33 (21.2052, 7.0268)
  point P34 (19.7999, 7.3415)
  point P35 (18.3807, 7.6524)
  point P36 (16.9489, 7.9585)
  point P37 (15.5058, 8.259)
  point P38 (14.0527, 8.5531)
  point P39 (12.5909, 8.8398)
  point P40 (11.1216, 9.1185)
  point P41 (9.6462, 9.3884)
  point P42 (8.1658, 9.6488)
  point P43 (6.6817, 9.8989)
  point P44 (5.1951, 10.138)
  point P45 (3.7071, 10.3656)
  point P46 (2.2189, 10.5811)
  point P47 (0.7317, 10.7838)
  point P48 (-0.7533, 10.9733)
  point P49 (-2.2351, 11.149)
  point P50 (-3.7126, 11.3105)
  point P51 (-5.1846, 11.4574)
  point P52 (-6.65, 11.5893)
  point P53 (-8.1078, 11.7058)
  point P54 (-9.5569, 11.8067)
  point P55 (-10.9963, 11.8916)
  point P56 (-12.4249, 11.9604)
  point P57 (-13.8416, 12.0129)
  point P58 (-15.2456, 12.0489)
  point P59 (-16.6357, 12.0682)
  point P60 (-18.0111, 12.0708)
  point P61 (-19.3706, 12.0567)
  point P62 (-20.7134, 12.0258)
  point P63 (-22.0386, 11.9782)
  point P64 (-23.3451, 11.914)
  point P65 (-24.6321, 11.8332)
  point P66 (-25.8986, 11.7359)
  point P67 (-27.1438, 11.6224)
  point P68 (-28.3668, 11.4928)
  point P69 (-29.5668, 11.3475)
  point P70 (-30.7428, 11.1865)
  point P71 (-31.8942, 11.0103)
  point P72 (-33.0199, 10.8192)
  point P73 (-34.1193, 10.6134)
  point P74 (-35.1916, 10.3935)
  point P75 (-36.236, 10.1598)
  point P76 (-37.2518, 9.9128)
  point P77 (-38.2382, 9.6529)
  point P78 (-39.1946, 9.3806)
  point P79 (-40.1201, 9.0964)
  point P80 (-41.0143, 8.8009)
  point P81 (-41.8763, 8.4946)
  point P82 (-42.7056, 8.1782)
  point P83 (-43.5016, 7.8521)
  point P84 (-44.2637, 7.5172)
  point P85 (-44.9912, 7.1738)
  point P86 (-45.6836, 6.8229)
  point P87 (-46.3405, 6.4649)
  point P88 (-46.9612, 6.1006)
  point P89 (-47.5454, 5.7307)
  point P90 (-48.0924, 5.3559)
  point P91 (-48.6019, 4.977)
  point P92 (-49.0734, 4.5946)
  point P93 (-49.5066, 4.2094)
  point P94 (-49.9009, 3.8224)
  point P95 (-50.2562, 3.4341)
  point P96 (-50.572, 3.0453)
  point P97 (-50.848, 2.6569)
  point P98 (-51.0839, 2.2695)
  point P99 (-51.2794, 1.884)
  point P100 (-51.4343, 1.501)
  point P101 (-51.5483, 1.1214)
  point P102 (-51.6212, 0.7459)
  point P103 (-51.6529, 0.3752)
  point P104 (-51.6432, 0.0101)
  point P105 (-51.5919, -0.3488)
  point P106 (-51.4988, -0.7006)
  point P107 (-51.364, -1.0447)
  point P108 (-51.1873, -1.3804)
  point P109 (-50.9687, -1.707)
  point P110 (-50.7081, -2.0239)
  point P111 (-50.4055, -2.3304)
  point P112 (-50.061, -2.6259)
  point P113 (-49.6745, -2.9099)
  point P114 (-49.2461, -3.1816)
  point P115 (-48.776, -3.4407)
  point P116 (-48.2641, -3.6865)
  point P117 (-47.7107, -3.9186)
  point P118 (-47.1158, -4.1366)
  point P119 (-46.4797, -4.3399)
  point P120 (-45.8025, -4.5283)
  point P121 (-45.0844, -4.7014)
  point P122 (-44.3258, -4.8588)
  point P123 (-43.5268, -5.0002)
  point P124 (-42.6879, -5.1255)
  point P125 (-41.8092, -5.2344)
  point P126 (-40.8911, -5.3269)
  point P127 (-39.9341, -5.4027)
  point P128 (-38.9385, -5.4619)
  point P129 (-37.9048, -5.5044)
  point P130 (-36.8334, -5.5303)
  point P131 (-35.7249, -5.5397)
  point P132 (-34.5798, -5.5327)
  point P133 (-33.3986, -5.5095)
  point P134 (-32.182, -5.4704)
  point P135 (-30.9307, -5.4157)
  point P136 (-29.6453, -5.3458)
  point P137 (-28.3266, -5.261)
  point P138 (-26.9753, -5.1619)
  point P139 (-25.5924, -5.049)
  point P140 (-24.1786, -4.9229)
  point P141 (-22.735, -4.7842)
  point P142 (-21.2625, -4.6337)
  point P143 (-19.7621, -4.472)
  point P144 (-18.2351, -4.2999)
  point P145 (-16.6825, -4.1184)
  point P146 (-15.1056, -3.9282)
  point P147 (-13.5057, -3.7304)
  point P148 (-11.8843, -3.5259)
  point P149 (-10.2427, -3.3156)
  point P150 (-8.5824, -3.1007)
  point P151 (-6.9052, -2.8822)
  point P152 (-5.2127, -2.6612)
  point P153 (-3.5065, -2.4388)
  point P154 (-1.7887, -2.216)
  point P155 (-0.0611, -1.994)
  point P156 (1.6743, -1.774)
  point P157 (3.4154, -1.557)
  point P158 (5.16, -1.344)
  point P159 (6.906, -1.1362)
  point P160 (8.6509, -0.9346)
  point P161 (10.3924, -0.7401)
  point P162 (12.128, -0.5537)
  point P163 (13.8553, -0.3762)
  point P164 (15.5716, -0.2086)
  point P165 (17.2743, -0.0514)
  point P166 (18.9608, 0.0946)
  point P167 (20.6284, 0.2288)
  point P168 (22.2743, 0.3508)
  point P169 (23.8958, 0.4602)
  point P170 (25.4901, 0.5567)
  point P171 (27.0546, 0.6401)
  point P172 (28.5864, 0.7104)
  point P173 (30.083, 0.7676)
  point P174 (31.5415, 0.8118)
  point P175 (32.9595, 0.8434)
  point P176 (34.3343, 0.8627)
  point P177 (35.6636, 0.8703)
  point P178 (36.9449, 0.8666)
  point P179 (38.176, 0.8525)
  point P180 (39.3546, 0.8287)
  point P181 (40.4788, 0.7961)
  point P182 (41.5466, 0.7556)
  point P183 (42.5563, 0.7084)
  point P184 (43.5062, 0.6555)
  point P185 (44.3948, 0.5981)
  point P186 (45.2209, 0.5373)
  point P187 (45.9833, 0.4745)
  point P188 (46.6809, 0.4109)
  point P189 (47.313, 0.3477)
  point P190 (47.879, 0.2863)
  point P191 (48.3782, 0.2278)
  point P192 (48.8105, 0.1735)
  point P193 (49.1757, 0.1246)
  point P194 (49.4737, 0.0823)
  point P195 (49.7048, 0.0477)
  point P196 (49.8692, 0.0218)
  point P197 (49.9674, 0.0056)
  dimension "d3" = 101.6529
  dimension "d4" = 9
  dimension "d5" = 25.4133
  dimension "d7" = 28
  dimension "d8" = 3.3
  constraint horizontal L0
  constraint coincident A0.centre L1.start
  constraint parallel L0 L1
  constraint coincident L1.end A1.centre
  measures "d3" distance of S0.start P103
  measures "d4" diameter of A0
  measures "d5" horizontal distance of P103 A0.centre
  measures "d7" distance of A0.centre L1.end
  measures "d8" diameter of A1
extrude "Extrusion1" add sketch "Esquisse2" along normal blind 188
